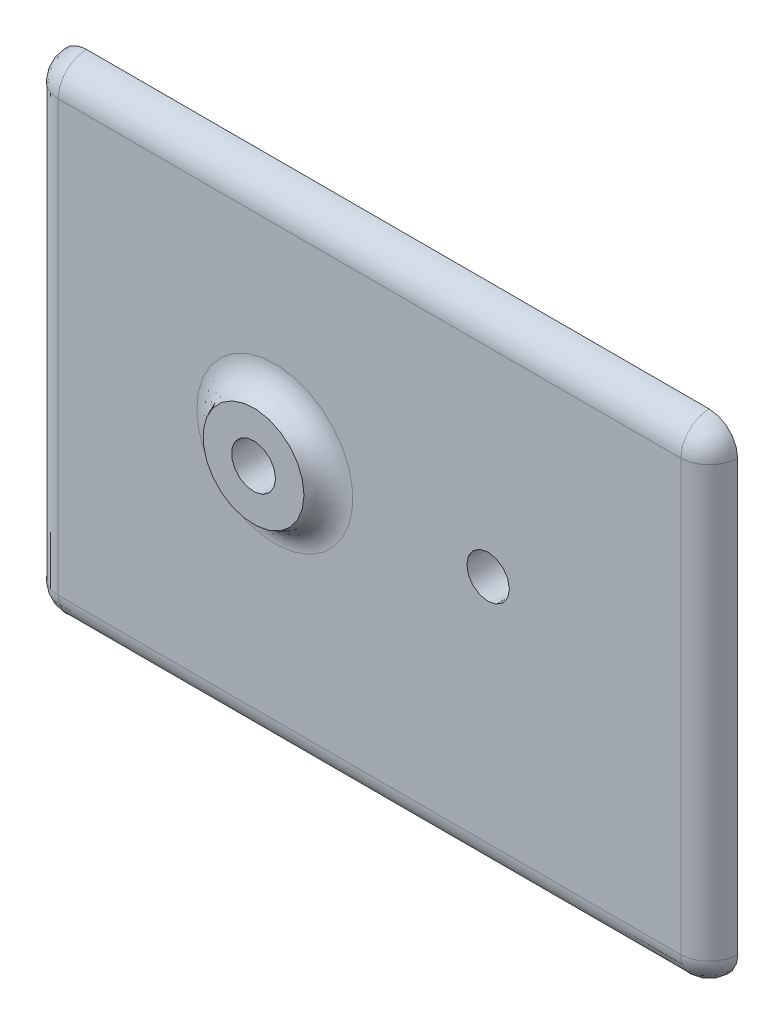
# Autodesk Inventor part: GehäuseBack
Saved by Autodesk Inventor 2014 (Build 180170000, 170)
## iProperties
Created: 2013-05-31
Part Number: GehäuseBack
Material: Generisch
Document SubType Name: Modeling
Designer: hanse
Density: 1 g/cm^3
Appearance: Vorgabe
Author: hanse
Autodesk Inventor part; units mm, degrees
ref_plane "YZ Plane" through (0, 0, 0) normal (1, 0, 0) x (0, 1, 0)
ref_plane "XZ Plane" through (0, 0, 0) normal (0, 1, 0) x (-1, 0, 0)
ref_plane "XY Plane" through (0, 0, 0) normal (0, 0, 1) x (1, 0, 0)
sketch "Skizze1" plane through (0, 0, 0) normal (0, 0, 1) x (1, 0, 0)
  line L0 (-21.8999, -15.1227) -> (-21.8999, 15.1227) projected
  line L1 (-21.8999, 15.1227) -> (21.8999, 15.1227) projected
  line L2 (21.8999, 15.1227) -> (21.8999, -15.1227) projected
  line L3 (21.8999, -15.1227) -> (-21.8999, -15.1227) projected
  line L4 (-21.8999, -17.1227) -> (21.8999, -17.1227) projected
  line L5 (23.8999, -15.1227) -> (23.8999, 15.1227) projected
  line L6 (21.8999, 17.1227) -> (-21.8999, 17.1227) projected
  line L7 (-23.8999, 15.1227) -> (-23.8999, -15.1227) projected
  circle A0 centre (8.3452, 1.1227) radius 1.5 projected
  circle A1 centre (-6.6548, 1.1227) radius 1.5 projected
  circle A2 centre (-6.6548, 1.1227) radius 1.55
  circle A3 centre (8.3452, 1.1227) radius 1.45
  arc A4 (-21.8999, 17.1227) -> (-23.8999, 15.1227) centre (-21.8999, 15.1227) ccw projected
  arc A5 (-23.8999, -15.1227) -> (-21.8999, -17.1227) centre (-21.8999, -15.1227) ccw projected
  arc A6 (21.8999, -17.1227) -> (23.8999, -15.1227) centre (21.8999, -15.1227) ccw projected
  arc A7 (23.8999, 15.1227) -> (21.8999, 17.1227) centre (21.8999, 15.1227) ccw projected
  point P0 (0, 0)
  dimension "d0" = 3.1
  dimension "d1" = 2.9
  constraints: 2 centre point, 2 coincident
  measures "d0" diameter of A2
  measures "d1" diameter of A3
extrude "Extrusion1" add sketch "Skizze1" along normal blind 2 contours L0 L1 L2 L3 | A5 L7 A4 L6 A7 L5 A6 L4
sketch "Skizze2" plane through (0, 0, 0) normal (0, 0, -1) x (-1, 0, 0)
  circle A0 centre (-8.3452, 1.1227) radius 1.5 projected
  circle A1 centre (-8.3452, 1.1227) radius 3.5
  point P0 (0, 0)
  dimension "d4" = 2
  constraints: 1 centre point, 1 coincident
  measures "d4" radial gap between concentric circles of A1 A0
extrude "Extrusion2" add sketch "Skizze2" along normal blind 3.5
fillet "Rundung1" radius 2 1 edges at (11.8452, 1.1227, 0)
fillet "Rundung2" radius 2 8 edges at (23.3141, 16.5369, 2) (0, 17.1227, 2) (-23.3141, 16.5369, 2) (-23.8999, 0, 2) (-23.3141, -16.5369, 2) (0, -17.1227, 2) (23.3141, -16.5369, 2) (23.8999, 0, 2)
sketch "Skizze3" plane through (0, 0, 2) normal (0, 0, 1) x (1, 0, 0)
  circle A0 centre (-6.6548, 1.1227) radius 1.55 projected
  circle A1 centre (-6.6548, 1.1227) radius 3.55
  point P0 (0, 0)
  dimension "d9" = 2
  constraints: 1 centre point, 1 coincident
  measures "d9" radial gap between concentric circles of A0 A1
extrude "Extrusion3" add sketch "Skizze3" along normal blind 1.5
fillet "Rundung3" radius 2 1 edges at (-10.2048, 1.1227, 2)
